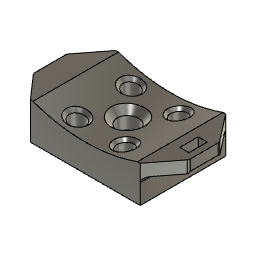
RGB_reader_support_rubberband v1 (Autodesk Fusion 360 design; units mm, degrees)
Autodesk Fusion 360 part; units mm, degrees
sketch "Sketch1" plane through (0, 0, 0) normal (0, 0, 1) x (1, 0, 0)
  line L0 (-18, -14) -> (18, -14)
  line L1 (18, -14) -> (18, 14)
  line L2 (18, 14) -> (-18, 14)
  line L3 (-18, 14) -> (-18, -14)
  line L4 (0, 35) -> (0, -60) construction
  line L5 (-65, 0) -> (75, 0) construction
  line L6 (-16, 12.1) -> (16, 12.1)
  line L7 (16, 12.1) -> (16, -12.1)
  line L8 (16, -12.1) -> (-16, -12.1)
  line L9 (-16, -12.1) -> (-16, 12.1)
  line L10 (0, 35) -> (0, -60) construction
  line L11 (-65, 0) -> (75, 0) construction
  line L12 (-4.4, 2.6) -> (4.4, 2.6)
  line L13 (4.4, 2.6) -> (4.4, -2.6)
  line L14 (4.4, -2.6) -> (-4.4, -2.6)
  line L15 (-4.4, -2.6) -> (-4.4, 2.6)
  line L16 (-5.75, 4.5) -> (5.75, 4.5)
  line L17 (5.75, 4.5) -> (5.75, -4.5)
  line L18 (5.75, -4.5) -> (-5.75, -4.5)
  line L19 (-5.75, -4.5) -> (-5.75, 4.5)
  line L20 (-16, -12.1) -> (-12, -12.1)
  line L21 (-12, -12.1) -> (-12, -7)
  line L22 (-12, -7) -> (-16, -7)
  line L23 (-16, -7) -> (-16, -12.1)
  line L24 (16, -12.1) -> (12, -12.1)
  line L25 (12, -12.1) -> (12, -7)
  line L26 (12, -7) -> (16, -7)
  line L27 (16, -7) -> (16, -12.1)
  line L28 (16, 12.1) -> (12, 12.1)
  line L29 (12, 12.1) -> (12, 7)
  line L30 (12, 7) -> (16, 7)
  line L31 (16, 7) -> (16, 12.1)
  line L32 (-16, 12.1) -> (-12, 12.1)
  line L33 (-12, 12.1) -> (-12, 7)
  line L34 (-12, 7) -> (-16, 7)
  line L35 (-16, 7) -> (-16, 12.1)
  dimension "d1" = 36
  dimension "d2" = 28
  dimension "d3" = 32
  dimension "d4" = 24.2
  dimension "d17" = 5.2
  dimension "d18" = 9
  dimension "d19" = 8.8
  dimension "d20" = 11.5
  constraint horizontal L0
  constraint vertical L1
  constraint horizontal L2
  constraint vertical L3
  constraint vertical L4
  constraint coincident origin L4
  constraint symmetric L1 L3 L4
  constraint horizontal L5
  constraint symmetric L0 L2 L5
  constraint horizontal L6
  constraint vertical L7
  constraint horizontal L8
  constraint vertical L9
  constraint symmetric L5 L6 L8
  constraint symmetric L4 L7 L9
  constraint vertical L10
  constraint coincident origin L10
  constraint horizontal L11
  constraint horizontal L12
  constraint vertical L13
  constraint horizontal L14
  constraint vertical L15
  constraint horizontal L16
  constraint vertical L17
  constraint horizontal L18
  constraint vertical L19
  constraint symmetric L5 L16 L18
  constraint symmetric L5 L12 L14
  constraint symmetric L10 L13 L15
  constraint symmetric L10 L17 L19
  constraint horizontal L20
  constraint vertical L21
  constraint horizontal L22
  constraint vertical L23
  constraint horizontal L24
  constraint vertical L25
  constraint horizontal L26
  constraint vertical L27
  constraint horizontal L28
  constraint vertical L29
  constraint horizontal L30
  constraint vertical L31
  constraint horizontal L32
  constraint vertical L33
  constraint horizontal L34
  constraint vertical L35
  measures "d1" distance of L0.start L0.end
  measures "d2" distance of L0.start L2.end
  measures "d3" distance of L6.start L6.end
  measures "d4" distance of L6.start L8.end
  measures "d17" distance of L12.end L13.end
  measures "d18" distance of L16.end L17.end
  measures "d19" distance of L12.start L12.end
  measures "d20" distance of L16.start L16.end
sketch "Sketch2" plane through (0, 0, 0) normal (0, 0, 1) x (1, 0, 0)
  line L0 (-18, 14) -> (-18, -14)
  line L1 (-65, 0) -> (75, 0) construction
  circle A0 centre (-7.8, -8.8) radius 2.625
  circle A1 centre (-7.8, 8.8) radius 2.625
  line L2 (-18, -14) -> (18, -14)
  circle A2 centre (7.8, -8.8) radius 2.625
  line L3 (0, 35) -> (0, -60) construction
  line L4 (18, -14) -> (18, 14)
  circle A3 centre (7.8, 8.8) radius 2.625
  line L5 (18, 14) -> (-18, 14)
  circle A4 centre (0, 0) radius 3.5
  dimension "d9" = 36
  dimension "d10" = 28
  dimension "d13" = 5.25
  dimension "d14" = 8.8
  dimension "d15" = 7.8
  dimension "d21" = 7
  constraint horizontal L2
  constraint vertical L4
  constraint horizontal L5
  constraint vertical L0
  constraint coincident A4.centre origin
  constraint vertical L3
  constraint coincident A4.centre L3
  constraint symmetric L0 L3 L4
  constraint horizontal L1
  constraint symmetric L1 L2 L5
  constraint equal A1 A3
  constraint equal A1 A2
  constraint equal A0 A1
  constraint symmetric A1 L3 A3
  constraint symmetric A0 A2 L3
  constraint symmetric L1 A0 A1
  constraint symmetric L1 A2 A3
  measures "d9" distance of L0.end L2.end
  measures "d10" distance of L0.start L0.end
  measures "d13" diameter of A1
  measures "d14" distance of A1.centre L1
  measures "d15" distance of A1.centre L3
  measures "d21" diameter of A4
extrude "Extrude1" add sketch "Sketch2" along normal blind 9
extrude "Extrude2" add sketch "Sketch1" against normal blind 1.9
sketch "Sketch4" plane through (0, -14, 0) normal (0, -1, 0) x (1, 0, 0)
  line L0 (18, -1.9) -> (18, 9)
  line L1 (18, 9) -> (-18, 9)
  line L2 (-18, 9) -> (-18, -1.9)
  line L3 (-18, -1.9) -> (18, -1.9)
  circle A0 centre (0, 56.5) radius 50.5
  line L4 (16, 0) -> (-16, 0)
  dimension "d32" = 101
  dimension "d33" = 56.5
  measures "d32" diameter of A0
  measures "d33" distance of A0.centre L4
extrude "Extrude4" cut sketch "Sketch4" against normal blind 36 contours L1 A0 picked at (3.4737, 8.3623)
extrude "Extrude5" add sketch "Sketch1" against normal up to surface (1.9 mm away) contours L6 L9 L32 L33 L34 L35 | L6 L7 L28 L29 L30 L31 | L8 L9 L20 L21 L22 L23 | L7 L8 L24 L25 L26 L27
extrude "Extrude6" add sketch "Sketch1" against normal blind 3 contours L0 L1 L2 L3
chamfer "Chamfer4" distance 1 angle 45 4 edges at (5.175, 8.8, 6.2659) (5.175, -8.8, 6.2659) (-10.425, 8.8, 7.0878) (-10.425, -8.8, 7.0878)
chamfer "Chamfer5" distance 2 angle 45 1 edges at (-3.5, 0, 6.1214)
chamfer "Chamfer6" distance 0.8 angle 45 2 edges at (0, 2.6, 0) (0, -2.6, 0)
sketch "Sketch5" plane through (0, 0, 9) normal (0, 0, 1) x (-1, 0, 0)
  line L0 (-25, -5) -> (-25, 5)
  line L1 (-18, 5) -> (-18, -5)
  line L2 (-20, -3) -> (-23, -3)
  line L3 (-23, -3) -> (-23, 3)
  line L4 (-23, 3) -> (-20, 3)
  line L5 (-20, 3) -> (-20, -3)
  line L6 (25, -5) -> (25, 6)
  line L7 (18, 6) -> (18, -5)
  line L8 (-18, 5) -> (-18, 14)
  line L9 (-18, 14) -> (-25, 5)
  line L10 (-18, -14) -> (-25, -5)
  line L11 (-18, -5) -> (-18, -14)
  line L12 (25, 6) -> (18, 14)
  line L13 (18, 14) -> (18, 6)
  line L14 (25, -5) -> (18, -14)
  line L15 (18, -14) -> (18, -5)
  constraint vertical L0
  constraint vertical L1
  constraint horizontal L2
  constraint vertical L3
  constraint horizontal L4
  constraint vertical L5
  constraint vertical L6
  constraint vertical L7
extrude "Extrude8" add sketch "Sketch5" against normal blind 4 contours L0 L1 L8 L9 L10 L11
extrude "Extrude9" add sketch "Sketch5" against normal blind 3 contours L6 L7 L12 L13 L14 L15
sketch "Sketch6" plane through (-25, 0, 0) normal (-1, 0, 0) x (0, -1, 0)
  line L0 (6, 9) -> (-5, 9)
  line L1 (-5, 9) -> (-5, 6)
  line L2 (-5, 6) -> (6, 6)
  line L3 (6, 6) -> (6, 9)
  line L4 (-3.1808, 6) -> (-0.0111, 6)
  line L5 (0, 0.95) -> (-0.0111, 6)
  spline S0 degree 5 poles (0, 0.95) (-0.1334, 0.95) (-0.3878, 0.9506) (-0.7325, 0.9531) (-1.1221, 0.9609) (-1.5162, 0.9845) (-1.8477, 1.0299) (-2.1474, 1.1048) (-2.4403, 1.2149) (-2.739, 1.3619) (-3.0363, 1.5408) (-3.3116, 1.7433) (-3.5382, 1.9603) (-3.6914, 2.1852) (-3.7552, 2.4168) (-3.7316, 2.6633) (-3.6368, 2.9384) (-3.4959, 3.2552) (-3.3373, 3.6216) (-3.1875, 4.0347) (-3.0656, 4.4742) (-2.9824, 4.9072) (-2.9422, 5.297) (-2.9435, 5.6108) (-2.9798, 5.8277) (-3.0406, 5.9469) (-3.0978, 5.9856) (-3.1402, 5.9974) (-3.1674, 6) (-3.1808, 6) knots 0 0 0 0 0 0 0.04 0.08 0.12 0.16 0.2 0.24 0.28 0.32 0.36 0.4 0.44 0.48 0.52 0.56 0.6 0.64 0.68 0.72 0.76 0.8 0.84 0.88 0.92 0.96 1 1 1 1 1 1
  line L6 (1, 0.95) -> (-1, 0.95)
  line L7 (-2.8, 6) -> (-3.5616, 6)
  point P0 (-2.4836, 1.2426)
  point P1 (-3.6899, 2.235)
  point P2 (-3.2995, 3.7375)
  point P3 (-2.9837, 5.7953)
  constraint coincident L2 L4.start
  constraint coincident L2 L4.end
  constraint midpoint L5.start L6
  constraint midpoint L4.start L7
  constraint coincident L4 L7.start
  constraint parallel L4 L7
revolve "Revolve2" add sketch "Sketch6" angle 180 about axis through (-25, 0, 0.95) along (0, -0.002205, -0.999998) contours L2 L4 L5 S0 L7
fillet "Fillet3" radius 0.5 2 edges at (-25, 3.7335, 2.5428) (-25, -3.7272, 2.44)
fillet "Fillet4" radius 1.5 2 edges at (18, 0, 5) (-18, 0, 6)
fillet "Fillet5" radius 0.5 2 edges at (23, 0, 5) (25, 0, 5)
fillet "Fillet5" radius 1.25 4 edges at (25, -5, 7) (25, 5, 7) (-25, 5, 7.5) (-25, -6, 7.5)
